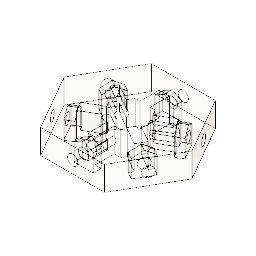
CapacitorJig2.7nF470pF (Autodesk Fusion 360 design; units mm, degrees)
Autodesk Fusion 360 part; units mm, degrees
note: some values were not read from the file. Chosen so that the rebuilt part matches the saved one: a direction; which face or edge a step refers to. Set by a fixed rule: which sketch regions a step uses.
sketch "Sketch1" plane through (0, 0, 0) normal (0, 0, 1) x (1, 0, 0)
  line L0 (-5.4993, 9.525) -> (-10.9985, 0)
  line L1 (-10.9985, 0) -> (-5.4993, -9.525)
  line L2 (-5.4993, -9.525) -> (5.4993, -9.525)
  line L3 (5.4993, -9.525) -> (10.9985, 0)
  line L4 (10.9985, 0) -> (5.4993, 9.525)
  line L5 (5.4993, 9.525) -> (-5.4993, 9.525)
  line L6 (-8.386, -14.525) -> (8.386, -14.525)
  line L7 (8.386, -14.525) -> (16.772, 0)
  line L8 (16.772, 0) -> (8.386, 14.525)
  line L9 (8.386, 14.525) -> (-8.386, 14.525)
  line L10 (-8.386, 14.525) -> (-16.772, 0)
  line L11 (-16.772, 0) -> (-8.386, -14.525)
  dimension "d1" = 19.05
  dimension "d2" = 5
  measures "d1" distance of L2 L5
extrude "Extrude1" add sketch "Sketch1" along normal blind 6.35
sketch "Sketch2" plane through (0, 0, 6.35) normal (0, 0, 1) x (-1, 0, 0)
  line L0 (5.4993, -9.525) -> (-5.4993, -9.525)
  line L1 (-5.4993, -9.525) -> (-10.9985, 0)
  line L2 (-10.9985, 0) -> (-5.4993, 9.525)
  line L3 (-5.4993, 9.525) -> (5.4993, 9.525)
  line L4 (5.4993, 9.525) -> (10.9985, 0)
  line L5 (10.9985, 0) -> (5.4993, -9.525)
  line L6 (16.772, 0) -> (8.386, 14.525)
  line L7 (8.386, 14.525) -> (-8.386, 14.525)
  line L8 (-8.386, 14.525) -> (-16.772, 0)
  line L9 (-16.772, 0) -> (-8.386, -14.525)
  line L10 (-8.386, -14.525) -> (8.386, -14.525)
  line L11 (8.386, -14.525) -> (16.772, 0)
  line L12 (1.35, -9.525) -> (1.35, -1.8187)
  line L13 (1.35, -1.8187) -> (7.7989, -5.5419)
  line L14 (0, 0) -> (8.2489, -4.7625)
  dimension "d5" = 1.35
  dimension "d24" = 0.9
  constraint perpendicular L10 L12
  constraint coincident L0 L12.start
  constraint coincident L5 L13.end
  constraint perpendicular L5 L13
  constraint coincident L14.start origin
  constraint midpoint L5 L14.end
  measures "d5" horizontal distance of L14.start L12.start
  measures "d24" distance of L13 L14
extrude "Extrude2" add sketch "Sketch2" against normal up to surface (6.35 mm away) contours L0 L5 L12 L13
mirror "Mirror1" about plane through (0, 0, 0) normal (1, 0, 0) of "Extrude2"
pattern_circular "C-Pattern4" count 3 over 360 about axis through (0, 0, 1.75) along (0, 0, 1) of "Extrude2", "Mirror1"
sketch "Sketch3" plane through (0, 14.525, 0) normal (0, 1, 0) x (-1, 0, 0)
  line L0 (-8.386, 0) -> (8.386, 0)
  line L1 (8.386, 0) -> (8.386, 6.35)
  line L2 (8.386, 6.35) -> (-8.386, 6.35)
  line L3 (-8.386, 6.35) -> (-8.386, 0)
  point P0 (0, 3.175)
  point P1 (8.386, 3.175)
  dimension "d21" = 3.175
  constraint midpoint L1 P1
  measures "d21" distance of L2 P0
hole "Hole1" at (0, 14.525, 3.175) direction (0, -1, 0) diameter 2.7 end through all
pattern_circular "C-Pattern2" count 3 over 360 about axis through (0, 0, 1.75) along (0, 0, 1) of "Hole1"
sketch "Sketch4" plane through (8.2489, -4.7625, 0) normal (-0.866025, 0.5, 0) x (-0.5, -0.866025, 0)
  line L0 (-1.35, 0) -> (1.35, 0)
  line L1 (1.35, 6.35) -> (-1.35, 6.35)
  line L2 (-2.5, 1.7316) -> (0, 0.2882)
  line L3 (0, 0.2882) -> (2.5, 1.7316)
  line L4 (2.5, 1.7316) -> (2.5, 4.6184)
  line L5 (2.5, 4.6184) -> (0, 6.0618)
  line L6 (0, 6.0618) -> (-2.5, 4.6184)
  line L7 (-2.5, 4.6184) -> (-2.5, 1.7316)
  line L8 (-2.5, 1.7316) -> (-2.5, 0)
  line L9 (-2.5, 0) -> (2.5, 0)
  line L10 (2.5, 0) -> (2.5, 1.7316)
  arc A0 (-1.35, 3.175) -> (1.35, 3.175) centre (0, 3.175) ccw
  line L11 (-1.35, 3.175) -> (-1.35, 0)
  line L12 (1.35, 0) -> (1.35, 3.175)
  arc A1 (1.35, 3.175) -> (-1.35, 3.175) centre (0, 3.175) ccw
  line L13 (1.35, 3.175) -> (1.35, 6.35)
  line L14 (-1.35, 6.35) -> (-1.35, 3.175)
  point P0 (0, 3.175)
  dimension "d15" = 5
  constraint vertical L7
  constraint parallel L7 L8
  constraint vertical L10
  constraint coincident origin L9
  measures "d15" distance of L4 L7
extrude "Extrude3" cut sketch "Sketch4" against normal blind 2.1 contours L0 L2 L3 L9 L11 L12 | L2 L8 L9 L11 | L3 L9 L10 L12 | L2 L3 A0 L11 L12 | L2 L6 L7 L11 L14 | L3 L4 L5 L12 L13 | L5 L6 A1 L13 L14
pattern_circular "C-Pattern3" count 6 over 360 about axis through (0, 0, 1.75) along (0, 0, 1) of "Extrude3"
sketch "Sketch5" plane through (0, 0, 0) normal (0, 0, 1) x (1, 0, 0)
  line L0 (2.5981, -4.5) -> (5.1962, 0)
  line L1 (5.1962, 0) -> (2.5981, 4.5)
  line L2 (2.5981, 4.5) -> (-2.5981, 4.5)
  line L3 (-2.5981, 4.5) -> (-5.1962, 0)
  line L4 (-5.1962, 0) -> (-2.5981, -4.5)
  line L5 (-2.5981, -4.5) -> (2.5981, -4.5)
  dimension "d22" = 9
  constraint horizontal L5
  measures "d22" distance of L2 L5
extrude "Extrude4" cut sketch "Sketch5" along normal through all
